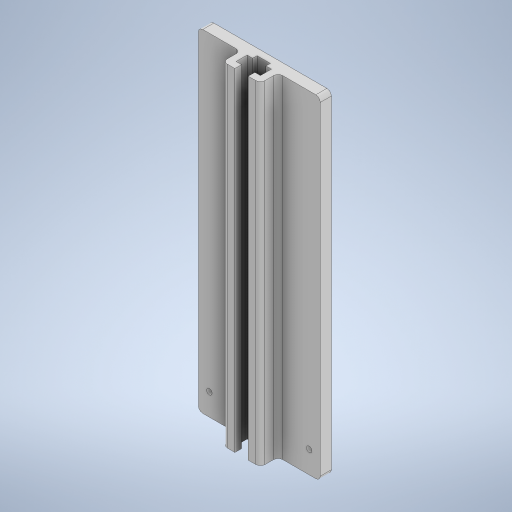
# Autodesk Inventor part: slide_part
Saved by Autodesk Inventor 2024.3 (Build 283343010, 343A)
## iProperties
Created: 2025-07-19
Part Number: slide_part
Material: 一般
Document SubType Name: Modeling
Designer: hikou
Density: 1 g/cm^3
Appearance: 既定
Author: hikou
Autodesk Inventor part; units mm, degrees
ref_plane "YZ Plane" through (0, 0, 0) normal (1, 0, 0) x (0, 1, 0)
ref_plane "XZ Plane" through (0, 0, 0) normal (0, 1, 0) x (-1, 0, 0)
ref_plane "XY Plane" through (0, 0, 0) normal (0, 0, 1) x (1, 0, 0)
sketch "スケッチ1" plane through (0, 0, 0) normal (0, 0, 1) x (1, 0, 0)
  line L0 (-27.5, -75) -> (27.5, -75)
  line L1 (27.5, -75) -> (27.5, 75)
  line L2 (27.5, 75) -> (-27.5, 75)
  line L3 (-27.5, 75) -> (-27.5, -75)
  line L4 (-27.5, -75) -> (27.5, 75) construction
  line L5 (27.5, -75) -> (-27.5, 75) construction
  point P0 (0, 0)
  dimension "d0" = 55
  dimension "d1" = 150
  constraints: 12 end point, 2 midpoint, 2 parallel, 1 horizontal, 1 perpendicular
  measures "d0" distance of L2.end L1.end
  measures "d1" distance of L1.end L0.end
extrude "押し出し1" add sketch "スケッチ1" along normal blind 5
sketch "スケッチ2" plane through (0, 0, 5) normal (0, 0, 1) x (1, 0, 0)
  line L0 (27.5, 75) -> (-27.5, 75) projected
  line L1 (-8.5, -75) -> (8.5, -75)
  line L2 (8.5, -75) -> (8.5, 75)
  line L3 (8.5, 75) -> (-8.5, 75)
  line L4 (-8.5, 75) -> (-8.5, -75)
  line L5 (-8.5, -75) -> (8.5, 75) construction
  line L6 (8.5, -75) -> (-8.5, 75) construction
  point P0 (0, 0)
  dimension "d4" = 17
  constraints: 12 end point, 2 midpoint, 2 parallel, 1 horizontal, 1 perpendicular, 1 point on line
  measures "d4" distance of L3.end L2.end
extrude "押し出し2" add sketch "スケッチ2" along normal blind 8
sketch "スケッチ3" plane through (-27.5, 75, 0) normal (0, 1, 0) x (1, 0, 0)
  line L0 (55, 0) -> (0, 0) projected
  line L1 (0, 0) -> (0, -5) projected
  line L2 (19, -5) -> (0, -5) projected
  line L3 (19, -5) -> (19, -13) projected
  line L4 (36, -13) -> (19, -13) projected
  line L5 (36, -5) -> (36, -13) projected
  line L6 (55, -5) -> (36, -5) projected
  line L7 (55, 0) -> (55, -5) projected
  line L8 (36, -5) -> (36, -13) projected
  line L9 (19, -5) -> (36, -5)
  line L10 (36, -5) -> (36, -10)
  line L11 (36, -10) -> (19, -10)
  line L12 (19, -10) -> (19, -5)
  line L13 (22, -5) -> (33, -5)
  line L14 (33, -5) -> (33, -10)
  line L15 (33, -10) -> (22, -10)
  line L16 (22, -10) -> (22, -5)
  line L17 (19, -13) -> (36, -13) projected
  line L18 (24.5, -10) -> (30.5, -10)
  line L19 (30.5, -10) -> (30.5, -13)
  line L20 (30.5, -13) -> (24.5, -13)
  line L21 (24.5, -13) -> (24.5, -10)
  line L22 (24.5, -5) -> (30.5, -5)
  line L23 (30.5, -5) -> (30.5, -3)
  line L24 (30.5, -3) -> (24.5, -3)
  line L25 (24.5, -3) -> (24.5, -5)
  point P0 (27.5, 0)
  dimension "d7" = 5
  dimension "d8" = 11
  dimension "d9" = 3
  dimension "d10" = 6
  dimension "d11" = 5.5
  dimension "d14" = 2
  constraints: 32 end point, 8 parallel, 6 point on line, 4 horizontal, 4 perpendicular
  measures "d7" distance of L9.end L10.end
  measures "d8" distance of L14.end L15.end
  measures "d9" distance between parallel lines of L16 L3
  measures "d10" distance of L19.end L20.end
  measures "d11" distance between parallel lines of L3 L21
  measures "d14" distance of L23.end L22.end
extrude "押し出し3" cut sketch "スケッチ3" against normal through all contours L14 L11 L16 L9 | L9 L25 L24 L23 | L4 L21 L11 L19
sketch "スケッチ4" plane through (0, 0, 0) normal (0, 0, -1) x (-1, 0, 0)
  line L0 (27.5, -75) -> (-27.5, -75) projected
  line L1 (-27.5, -75) -> (-27.5, 75) projected
  point P0 (0, 0)
  point P1 (-22.5, -65)
  point P2 (22.5, -65)
  dimension "d15" = 10
  dimension "d16" = 10
  dimension "d17" = 45
  dimension "d18" = 5
  measures "d15" distance from line of L0 point (-22.5, -65)
  measures "d16" distance from line of L0 point (22.5, -65)
  measures "d17" distance of point (22.5, -65) point (-22.5, -65)
  measures "d18" distance from line of L1 point (-22.5, -65)
hole "穴1" at (22.5, -65, 0) at (-22.5, -65, 0) direction (0, 0, 1) diameter 2.5 end through all
fillet "フィレット1" radius 2 8 edges at (-8.5, 0, 5) (8.5, 0, 5) (8.5, 0, 13) (-8.5, 0, 13) (27.5, -75, 2.5) (-27.5, -75, 2.5) (27.5, 75, 2.5) (-27.5, 75, 2.5)
